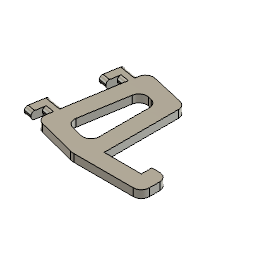
Skadis - Screen and pi500 mount (Autodesk Fusion 360 design; units mm, degrees)
Autodesk Fusion 360 part; units mm, degrees
sketch "Sketch1" plane through (0, 0, 0) normal (0, 1, 0) x (1, 0, 0)
  line L0 (201.1333, -44.3937) -> (206.1333, -44.3937)
  line L1 (211.1333, -49.3937) -> (211.1333, -55.8937)
  line L2 (206.1333, -60.8937) -> (201.1333, -60.8937)
  line L3 (201.1333, -60.8937) -> (201.1333, -44.3937)
  line L4 (201.1333, -60.8937) -> (178.1333, -60.8937)
  line L5 (178.1333, -60.8937) -> (178.1333, -50.8937)
  line L6 (178.1333, -50.8937) -> (201.1333, -50.8937)
  line L7 (201.1333, -50.8937) -> (201.1333, -60.8937)
  line L8 (178.1333, -60.8937) -> (168.1333, -60.8937)
  line L9 (168.1333, -60.8937) -> (168.1333, -0.8937)
  line L10 (168.1333, -0.8937) -> (178.1333, -0.8937)
  line L11 (178.1333, -0.8937) -> (178.1333, -60.8937)
  line L12 (178.1333, -0.8937) -> (154.0774, 4.6306)
  line L13 (168.1333, -60.8937) -> (143.5177, -54.5192)
  line L14 (148.0255, 0.5743) -> (139.8384, -48.862)
  arc A0 (154.0774, 4.6306) -> (148.0255, 0.5743) centre (152.9583, -0.2426) ccw
  arc A1 (139.8384, -48.862) -> (143.5177, -54.5192) centre (144.7712, -49.6789) ccw
  arc A2 (206.1333, -60.8937) -> (211.1333, -55.8937) centre (206.1333, -55.8937) ccw
  arc A3 (211.1333, -49.3937) -> (206.1333, -44.3937) centre (206.1333, -49.3937) ccw
  line L15 (161.8799, -48.9444) -> (154.8775, -47.1311)
  line L16 (156.1534, -11.5525) -> (151.1981, -41.4738)
  line L17 (164.2524, -7.9663) -> (162.2053, -7.4962)
  line L18 (168.1333, -12.8395) -> (168.1333, -44.1041)
  arc A4 (162.2053, -7.4962) -> (156.1534, -11.5525) centre (161.0862, -12.3694) ccw
  arc A5 (168.1333, -12.8395) -> (164.2524, -7.9663) centre (163.1333, -12.8395) ccw
  arc A6 (161.8799, -48.9444) -> (168.1333, -44.1041) centre (163.1333, -44.1041) ccw
  arc A7 (151.1981, -41.4738) -> (154.8775, -47.1311) centre (156.131, -42.2908) ccw
  point P0 (211.1333, -44.3937)
  point P1 (148.8944, 5.8208)
  point P2 (139.0913, -53.373)
  dimension "d18" = 10
  dimension "d19" = 16.5
  dimension "d20" = 23
  dimension "d21" = 10
  dimension "d22" = 10
  dimension "d23" = 60
  dimension "d25" = 30
  dimension "d26" = 30
  dimension "d27" = 60
  dimension "d28" = 75.482
  dimension "d29" = 95.115
  dimension "d30" = 5
  dimension "d32" = 5
  constraint horizontal L0
  constraint vertical L1
  constraint horizontal L2
  constraint vertical L3
  constraint horizontal L4
  constraint vertical L5
  constraint horizontal L6
  constraint vertical L7
  constraint horizontal L8
  constraint vertical L9
  constraint horizontal L10
  constraint vertical L11
  constraint coincident P1 L12
  constraint coincident P1 L14
  constraint tangent L12 A0
  constraint tangent L14 A0
  constraint coincident P2 L13
  constraint coincident P2 L14
  constraint tangent L13 A1
  constraint tangent L14 A1
  constraint equal A0 A1
  constraint tangent L1 A2
  constraint tangent L2 A2
  constraint equal A0 A2
  constraint coincident P0 L0
  constraint coincident P0 L1
  constraint tangent L0 A3
  constraint tangent L1 A3
  constraint equal A0 A3
  constraint tangent L16 A4
  constraint tangent L17 A4
  constraint tangent L17 A5
  constraint tangent L18 A5
  constraint equal A4 A5
  constraint tangent L15 A6
  constraint tangent L18 A6
  constraint equal A4 A6
  constraint tangent L15 A7
  constraint tangent L16 A7
  constraint equal A4 A7
  measures "d18" distance of L0.start P0
  measures "d19" distance of L0.start L2.end
  measures "d20" distance of L2.end L4.end
  measures "d21" distance of L2.end L6.end
  measures "d22" distance of L4.end L8.end
  measures "d23" distance of L4.end L10.end
  measures "d25" distance of L10.end P1
  measures "d26" distance of L8.end P2
  measures "d27" distance of P1 P2
  measures "d28" angle of L9 L13
  measures "d29" angle of L13 L14
  measures "d30" radius of A0
  measures "d32" radius of A4
extrude "Extrude1" add sketch "Sketch1" along normal blind 4.8 contours L0 L1 L2 L3 L7 A2 A3 | L3 L4 L5 L6 L7 L11 | L5 L8 L9 L10 L11 L18 | L9 L10 L12 L13 L14 A0 A1 L15 L16 L17 A4 A5 A6 A7
fillet "Fillet1" radius 5 1 edges at (178.1333, 2.4, 0.8937)
fillet "Fillet2" radius 10 1 edges at (168.1333, 2.4, 60.8937)
sketch "Sketch2" plane through (143.9815, 0, 23.8448) normal (-0.986562, 0, -0.163385) x (-0.163385, 0, 0.986562)
  line L0 (-24.7517, 0) -> (25.358, 0)
  line L1 (25.358, 0) -> (25.358, 4.8)
  line L2 (25.358, 4.8) -> (-24.7517, 4.8)
  line L3 (-24.7517, 4.8) -> (-24.7517, 0)
  line L4 (-22.442, 0) -> (-12.942, 0)
  line L5 (-10.942, 2) -> (-10.942, 2.8)
  line L6 (-12.942, 4.8) -> (-22.442, 4.8)
  line L7 (-24.442, 2.8) -> (-24.442, 2)
  arc A0 (-22.442, 4.8) -> (-24.442, 2.8) centre (-22.442, 2.8) ccw
  arc A1 (-24.442, 2) -> (-22.442, 0) centre (-22.442, 2) ccw
  arc A2 (-10.942, 2.8) -> (-12.942, 4.8) centre (-12.942, 2.8) ccw
  arc A3 (-12.942, 0) -> (-10.942, 2) centre (-12.942, 2) ccw
  line L8 (17.858, 0) -> (27.358, 0)
  line L9 (29.358, 2) -> (29.358, 2.8)
  line L10 (27.358, 4.8) -> (17.858, 4.8)
  line L11 (15.858, 2.8) -> (15.858, 2)
  arc A4 (15.858, 2) -> (17.858, 0) centre (17.858, 2) ccw
  arc A5 (17.858, 4.8) -> (15.858, 2.8) centre (17.858, 2.8) ccw
  arc A6 (29.358, 2.8) -> (27.358, 4.8) centre (27.358, 2.8) ccw
  arc A7 (27.358, 0) -> (29.358, 2) centre (27.358, 2) ccw
  line L12 (-17.142, 4.8) -> (-17.142, 0)
  line L13 (23.158, 4.8) -> (23.158, 0)
  point P0 (-24.442, 0)
  point P1 (-10.942, 0)
  point P2 (-24.442, 4.8)
  point P3 (15.858, 0)
  point P4 (29.358, 0)
  point P5 (15.858, 4.8)
  dimension "d39" = 13.5
  dimension "d40" = 4.8
  dimension "d41" = 2
  dimension "d42" = 13.5
  dimension "d43" = 4.8
  dimension "d44" = 2
  dimension "d45" = 53.8
  dimension "d49" = 4
  dimension "d50" = 7.3
  dimension "d51" = 7.3
  dimension "d56" = 6.2
  constraint horizontal L4
  constraint vertical L5
  constraint horizontal L6
  constraint vertical L7
  constraint coincident L0 P0
  constraint coincident P2 L6
  constraint coincident P2 L7
  constraint tangent L6 A0
  constraint tangent L7 A0
  constraint coincident P0 L4
  constraint coincident P0 L7
  constraint tangent L4 A1
  constraint tangent L7 A1
  constraint equal A0 A1
  constraint tangent L5 A2
  constraint tangent L6 A2
  constraint equal A0 A2
  constraint coincident P1 L4
  constraint coincident P1 L5
  constraint tangent L4 A3
  constraint tangent L5 A3
  constraint equal A0 A3
  constraint horizontal L8
  constraint vertical L9
  constraint horizontal L10
  constraint vertical L11
  constraint coincident L0 P3
  constraint coincident P3 L8
  constraint coincident P3 L11
  constraint tangent L8 A4
  constraint tangent L11 A4
  constraint coincident P5 L10
  constraint coincident P5 L11
  constraint tangent L10 A5
  constraint tangent L11 A5
  constraint equal A4 A5
  constraint tangent L9 A6
  constraint tangent L10 A6
  constraint equal A4 A6
  constraint coincident P4 L8
  constraint coincident P4 L9
  constraint tangent L8 A7
  constraint tangent L9 A7
  constraint equal A4 A7
  constraint coincident L6 L12.start
  constraint perpendicular L6 L12
  constraint coincident L0 L12.end
  constraint coincident L10 L13.start
  constraint perpendicular L10 L13
  constraint coincident L0 L13.end
  measures "d39" distance of P0 P1
  measures "d40" distance of P0 P2
  measures "d41" radius of A0
  measures "d42" distance of P3 P4
  measures "d43" distance of P3 P5
  measures "d44" radius of A4
  measures "d45" distance of L7 L9
  measures "d49" distance of L1 L9
  measures "d50" distance of L7 L12
  measures "d51" distance of L11 L13
  measures "d56" distance of L9 L13
extrude "Extrude2" add sketch "Sketch2" along normal blind 10.4 contours L0 L2 L4 L6 L7 A0 A1 L12 | L0 L2 L4 L5 L6 A2 A3 L12 | L0 L2 L8 L10 L11 A4 A5 L13
extrude "Extrude3" cut sketch "Sketch2" along normal blind 5.4 contours L0 L2 L4 L5 L6 A2 A3 L12
extrude "Extrude4" cut sketch "Sketch2" along normal blind 5.4 contours L0 L1 L2 L8 L10 L13
sketch "Sketch3" plane through (-3.7837, 0, 22.8468) normal (-0.163385, 0, 0.986562) x (0.986562, 0, 0.163385)
  line L0 (145.9426, 0) -> (145.9426, 4.8)
  line L1 (145.9426, 4.8) -> (135.5426, 4.8)
  line L2 (135.5426, 4.8) -> (135.5426, 0)
  line L3 (135.5426, 0) -> (145.9426, 0)
  line L4 (135.5426, 0) -> (140.5426, 0)
  line L5 (140.5426, 0) -> (140.5426, 4.8)
  line L6 (140.5426, 4.8) -> (135.5426, 4.8)
  line L7 (135.5426, 4.8) -> (135.5426, 0)
  dimension "d57" = 5
  dimension "d58" = 4.8
  constraint horizontal L4
  constraint vertical L5
  constraint horizontal L6
  constraint vertical L7
  constraint coincident L2.end L3.start
  measures "d57" distance of L2.end L4.end
  measures "d58" distance of L2.end L1.end
extrude "Extrude5" add sketch "Sketch3" along normal blind 6.2 contours L1 L2 L3 L4 L5 L6 L7
fillet "Fillet4" radius 2 2 edges at (131.391, 4.8, 51.5175) (131.391, 0, 51.5175)
fillet "Fillet5" radius 2 4 edges at (144.1185, 4.8, 6.4919) (144.1185, 0, 6.4919) (137.5341, 4.8, 46.2504) (137.5341, 0, 46.2504)
equation "d47 = 5.4 mm + 5 mm"
